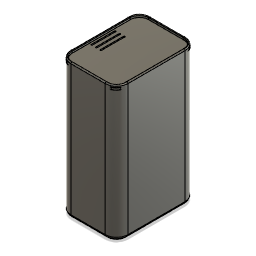
CableOrginiser_Type_4 v2 (Autodesk Fusion 360 design; units mm, degrees)
Autodesk Fusion 360 part; units mm, degrees
note: some values were not read from the file. Set by a fixed rule: which sketch regions a step uses.
sketch "Sketch1" plane through (0, 0, 0) normal (0, 1, 0) x (1, 0, 0) in component "BodyComponent"
  line L0 (0, 0) -> (50, 0)
  line L1 (50, 0) -> (50, 70)
  line L2 (50, 70) -> (0, 70)
  line L3 (0, 70) -> (0, 0)
  line L4 (0, 0) -> (1.5, 0) construction
  line L5 (1.5, 0) -> (1.5, 1.5) construction
  line L6 (1.5, 1.5) -> (0, 1.5) construction
  line L7 (0, 1.5) -> (0, 0) construction
  line L8 (1.5, 1.5) -> (48.5, 1.5)
  line L9 (48.5, 1.5) -> (48.5, 68.5)
  line L10 (48.5, 68.5) -> (1.5, 68.5)
  line L11 (1.5, 68.5) -> (1.5, 1.5)
  dimension "d1" = 50
  dimension "d2" = 70
  dimension "d3" = 1.5
  dimension "d4" = 1.5
  dimension "d5" = 47
  dimension "d6" = 67
  constraint horizontal L0
  constraint vertical L1
  constraint horizontal L2
  constraint vertical L3
  constraint coincident L0.start L3.end
  constraint horizontal L4
  constraint vertical L5
  constraint horizontal L6
  constraint vertical L7
  constraint horizontal L8
  constraint vertical L9
  constraint horizontal L10
  constraint vertical L11
  measures "d1" distance of L0.start L0.end
  measures "d2" distance of L0.start L2.end
  measures "d3" distance of L0.start L4.end
  measures "d4" distance of L0.start L6.end
  measures "d5" distance of L5.end L8.end
  measures "d6" distance of L5.end L10.end
extrude "Extrude1" add sketch "Sketch1" against normal blind 1.5 contours L0 L1 L2 L3 | L8 L9 L10 L11 makes body 1 in component "BodyComponent"
extrude "Extrude2" add sketch "Sketch1" along normal blind 118 bodies 1 in component "BodyComponent"
fillet "Fillet1" radius 8 4 edges at (1.5, 59, -68.5) (1.5, 59, -1.5) (48.5, 59, -1.5) (48.5, 59, -68.5) on bodies 1 in component "BodyComponent"
fillet "Fillet2" radius 10 4 edges at (0, 58.25, 0) (0, 58.25, -70) (50, 58.25, -70) (50, 58.25, 0) on bodies 1 in component "BodyComponent"
fillet "Fillet3" radius 3 8 edges at (1.5, 0, -35) (3.8431, 0, -3.8431) (25, 0, -1.5) (46.1569, 0, -3.8431) (48.5, 0, -35) (46.1569, 0, -66.1569) (25, 0, -68.5) (3.8431, 0, -66.1569) on bodies 1 in component "BodyComponent"
chamfer "Chamfer2" distance 3 angle 45 8 edges at (2.9289, -1.5, -2.9289) (0, -1.5, -35) (2.9289, -1.5, -67.0711) (25, -1.5, -70) (47.0711, -1.5, -67.0711) (50, -1.5, -35) (47.0711, -1.5, -2.9289) (25, -1.5, 0) on bodies 1 in component "BodyComponent"
fillet "Fillet11" radius 2 16 edges at (0, 1.5, -35) (2.9289, 1.5, -67.0711) (25, 1.5, -70) (47.0711, 1.5, -67.0711) (50, 1.5, -35) (47.0711, 1.5, -2.9289) (25, 1.5, 0) (2.9289, 1.5, -2.9289) (47, -1.5, -35) (44.9497, -1.5, -64.9497) (25, -1.5, -67) (5.0503, -1.5, -64.9497) (3, -1.5, -35) (5.0503, -1.5, -5.0503) (25, -1.5, -3) (44.9497, -1.5, -5.0503) on bodies 1 in component "BodyComponent"
sketch "Sketch3" plane through (0, 0, 0) normal (-1, 0, 0) x (0, 0, 1) in component "BodyComponent"
  line L0 (-69, 114) -> (-1, 114)
  line L1 (-1, 114) -> (-1, 116)
  line L2 (-1, 116) -> (-69, 116)
  line L3 (-69, 116) -> (-69, 114)
  line L4 (-60, 118) -> (-60, 2.3284)
  line L5 (-10, 2.3284) -> (-10, 118)
  line L6 (-10, 118) -> (-60, 118)
  line L7 (-35, 118) -> (-35, 116)
  line L8 (-60, 2.3284) -> (-10, 2.3284)
  dimension "d27" = 68
  dimension "d28" = 2
  dimension "d79" = 2
  constraint horizontal L0
  constraint vertical L1
  constraint horizontal L2
  constraint vertical L3
  constraint midpoint L2 L7.end
  constraint midpoint L6 L7.start
  constraint perpendicular L6 L7
  measures "d27" distance of L0.start L0.end
  measures "d28" distance of L0.start L2.end
  measures "d79" distance of L7.start L7.end
extrude "Extrude4" cut sketch "Sketch3" against normal blind 48.5 contours L0 L2 L3 L4 | L0 L2 L4 L5 | L0 L1 L2 L5 bodies 1 in component "BodyComponent"
sketch "Sketch2" plane through (0, 0, 0) normal (-1, 0, 0) x (0, 0, 1) in component "LidComponent"
  line L0 (-68.9, 114.2) -> (-1.1, 114.2)
  line L1 (-1.1, 114.2) -> (-1.1, 115.8)
  line L2 (-1.1, 115.8) -> (-68.9, 115.8)
  line L3 (-60, 114) -> (-60, 2.3284)
  line L4 (-10, 2.3284) -> (-10, 114)
  line L5 (-10, 114) -> (-60, 114)
  line L6 (-68.9, 115.8) -> (-68.9, 114.2)
  line L7 (-35, 114) -> (-35, 114.2)
  line L8 (-60, 2.3284) -> (-10, 2.3284)
  point P0 (-35, 114.2)
  dimension "d33" = 67.8
  dimension "d34" = 1.6
  dimension "d80" = 0.2
  constraint horizontal L0
  constraint vertical L1
  constraint horizontal L2
  constraint perpendicular L0 L6
  constraint midpoint L5 L7.start
  constraint vertical L7
  constraint midpoint L0 P0
  constraint coincident P0 L7.end
  measures "d33" distance of L0.start L0.end
  measures "d34" distance of L0.start L2.end
  measures "d80" distance of L7.start P0
extrude "Extrude1'" add sketch "Sketch2" against normal blind 48.5 separate body contours L0 L1 L2 L6 makes body 2 in component "LidComponent"
sketch "Sketch3 (2)" plane through (0, 115.8, 0) normal (0, 1, 0) x (-1, 0, 0) in component "LidComponent"
  line L0 (0, -1.1) -> (-48.5, -1.1)
  line L1 (-48.5, -1.1) -> (-48.5, -68.9)
  line L2 (0, -35) -> (-3, -35)
  line L3 (-3, -35) -> (-3, -45)
  line L4 (-3, -45) -> (-4, -45)
  line L5 (-4, -45) -> (-4, -25)
  line L6 (-4, -25) -> (-3, -25)
  line L7 (-3, -25) -> (-3, -45)
  line L8 (-4, -35) -> (-7, -35)
  line L9 (-7, -35) -> (-7, -45)
  line L10 (-7, -45) -> (-8, -45)
  line L11 (-8, -45) -> (-8, -25)
  line L12 (-8, -25) -> (-7, -25)
  line L13 (-7, -25) -> (-7, -45)
  line L14 (-8, -35) -> (-11, -35)
  line L15 (-11, -35) -> (-11, -45)
  line L16 (-11, -45) -> (-12, -45)
  line L17 (-12, -45) -> (-12, -25)
  line L18 (-12, -25) -> (-11, -25)
  line L19 (-11, -25) -> (-11, -45)
  line L20 (0, -68.9) -> (0, -1.1)
  line L21 (-48.5, -68.9) -> (0, -68.9)
  dimension "d45" = 3
  dimension "d46" = 10
  dimension "d47" = 1
  dimension "d48" = 20
  dimension "d49" = 3
  dimension "d50" = 10
  dimension "d51" = 1
  dimension "d52" = 20
  dimension "d53" = 3
  dimension "d54" = 10
  dimension "d55" = 1
  dimension "d56" = 20
  constraint perpendicular L2 L3
  constraint horizontal L4
  constraint vertical L5
  constraint horizontal L6
  constraint vertical L7
  constraint midpoint L5 L8.start
  constraint perpendicular L5 L8
  constraint perpendicular L8 L9
  constraint horizontal L10
  constraint vertical L11
  constraint horizontal L12
  constraint vertical L13
  constraint midpoint L11 L14.start
  constraint perpendicular L11 L14
  constraint perpendicular L14 L15
  constraint horizontal L16
  constraint vertical L17
  constraint horizontal L18
  constraint vertical L19
  constraint midpoint L2.start L20
  constraint perpendicular L2 L20
  measures "d45" distance of L2.start L2.end
  measures "d46" distance of L2.end L3.end
  measures "d47" distance of L3.end L4.end
  measures "d48" distance of L3.end L6.end
  measures "d49" distance of L8.start L8.end
  measures "d50" distance of L8.end L9.end
  measures "d51" distance of L9.end L10.end
  measures "d52" distance of L9.end L12.end
  measures "d53" distance of L14.start L14.end
  measures "d54" distance of L14.end L15.end
  measures "d55" distance of L15.end L16.end
  measures "d56" distance of L15.end L18.end
extrude "Extrude4'" cut sketch "Sketch3 (2)" against normal blind 1 contours L3 L4 L5 L6 L7 | L9 L10 L11 L12 L13 | L15 L16 L17 L18 L19 bodies 2 in component "LidComponent"
fillet "Fillet5" radius 8 2 edges at (0, 115, -1.1) (0, 115, -68.9) on bodies 2 in component "LidComponent"
fillet "Fillet6" radius 5 2 edges at (48.5, 115, -1.1) (48.5, 115, -68.9) on bodies 2 in component "LidComponent"
fillet "Fillet6'" radius 1 8 edges at (47.0711, 118, -2.9289) (50, 118, -35) (47.0711, 118, -67.0711) (25, 118, -70) (2.9289, 118, -67.0711) (0, 118, -35) (2.9289, 118, -2.9289) (25, 118, 0) on bodies 1 in component "BodyComponent"
fillet "Fillet7" radius 1 12 edges at (3.5, 114.8, -45) (3.5, 115.8, -45) (7.5, 114.8, -45) (7.5, 115.8, -45) (11.5, 114.8, -45) (11.5, 115.8, -45) (11.5, 114.8, -25) (11.5, 115.8, -25) (3.5, 114.8, -25) (3.5, 115.8, -25) (7.5, 114.8, -25) (7.5, 115.8, -25) on bodies 2 in component "LidComponent"
fillet "Fillet7'" radius 0.5 8 edges at (3.8431, 118, -66.1569) (25, 118, -68.5) (46.1569, 118, -66.1569) (48.5, 118, -35) (46.1569, 118, -3.8431) (25, 118, -1.5) (3.8431, 118, -3.8431) (1.5, 118, -35) on bodies 1 in component "BodyComponent"
component "BodyComponent" placed x (1, 0, 0) y (0, 1, 0) z (0, 0, 1) at (0, 0, 0)
component "LidComponent" placed x (1, 0, 0) y (0, 1, 0) z (0, 0, 1) at (0, 0, 0)
equation "d2 = 35 mm * 2"
equation "d5 = 48.500 mm - 1.5 mm"
